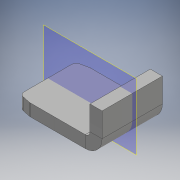
# Autodesk Inventor part: hage
Saved by Autodesk Inventor 2018 (Build 220112000, 112)
## iProperties
Created: 2019-09-30
Part Number: hage
Material: Steel
Document SubType Name: Sheet Metal
Designer: gust3763
Density: 7.85 g/cm^3
Sheet Metal Rule: Default_mm
Appearance: Light Gray
Mass: 86.5098 g
Surface Area: 39.7038 cm^2
Volume: 11.0204 cm^3
Author: gust3763
Autodesk Inventor part; units mm, degrees
ref_plane "YZ Plane" through (0, 0, 0) normal (1, 0, 0) x (0, 1, 0)
ref_plane "XZ Plane" through (0, 0, 0) normal (0, 1, 0) x (-1, 0, 0)
ref_plane "XY Plane" through (0, 0, 0) normal (0, 0, 1) x (1, 0, 0)
sketch "Sketch1" plane through (0, 0, 0) normal (0, 0, 1) x (1, 0, 0)
  line L0 (4.3681, -1.3047) -> (34.1579, -1.3047)
  line L1 (34.1579, -1.3047) -> (34.1579, 23.6953)
  line L2 (34.1579, 23.6953) -> (4.3681, 23.6953)
  line L3 (-0.8421, 21.0129) -> (-0.8421, 1.3776)
  line L4 (3.9523, 23.6516) -> (0.7421, 22.9692)
  line L5 (3.9523, -1.261) -> (0.7421, -0.5787)
  line L6 (4.1579, 23.6953) -> (4.1579, -1.3047) construction
  arc A0 (0.7421, 22.9692) -> (-0.8421, 21.0129) centre (1.1579, 21.0129) ccw
  arc A1 (-0.8421, 1.3776) -> (0.7421, -0.5787) centre (1.1579, 1.3776) ccw
  arc A2 (4.3681, 23.6953) -> (3.9523, 23.6516) centre (4.3681, 21.6953) ccw
  arc A3 (3.9523, -1.261) -> (4.3681, -1.3047) centre (4.3681, 0.6953) ccw
  point P0 (0, 0)
  point P1 (-0.8421, 22.6325)
  point P2 (-0.8421, -0.242)
  dimension "d3" = 12
  dimension "d4" = 25
  dimension "d5" = 12
  dimension "d7" = 35
  dimension "d8" = 5
  dimension "d20" = 2
  measures "d3" angle of L0 L5
  measures "d4" distance between parallel lines of L0 L2
  measures "d5" angle of L4 L2
  measures "d7" distance between parallel lines of L1 L3
  measures "d8" distance between parallel lines of L3 L6
  measures "d20" radius of A0
extrude "Plate1" add sketch "Sketch1" along normal blind 5
sketch "Sketch2" plane through (29.1579, 23.6953, 0) normal (1, 0, 0) x (0, 1, 0)
  line L0 (-25, 0) -> (0, 0)
  line L1 (0, 0) -> (0, 17)
  line L2 (0, 17) -> (-25, 17)
  line L3 (-25, 17) -> (-25, 0)
  constraints: 6 end point, 1 horizontal, 1 perpendicular, 1 vertical
edge flange "Flange1" height 12 angle 90 thickness 5 bend radius 2 thickness toward (1, 0, 0) relief straight relief width 5 relief depth 2.5 edges at (34.1579, 11.1953, 5) wall of the first edge with corners at (29.1579, -1.3047, 0) (29.1579, 23.6953, 0) (29.1579, 23.6953, 17) (29.1579, -1.3047, 17)
bend "Bend1"
corner "Corner1"
ref_plane "midtplan" through (4.3681, 11.1953, 5) normal (0, 1, 0) x (1, 0, 0)
equation "\"d3\" = d5"
equation "\"d9\" = Thickness"
equation "\"d10\" = BendReliefWidth"
equation "\"d11\" = BendReliefDepth"
equation "\"d12\" = MinimumRemnant"
equation "\"d13\" = TransitionRadius"
equation "\"d16\" = BendRadius"
equation "\"d17\" = CornerReliefSize"
equation "\"d18\" = GapSize"
equation "\"d19\" = JacobiRadiusSize"
equation "\"BendReliefWidth\" = Thickness"
equation "\"BendReliefDepth\" = 0.5 * Thickness"
equation "\"TransitionRadius\" = BendRadius"
equation "\"JacobiRadiusSize\" = BendRadius"
equation "\"GapSize\" = Thickness"
equation "\"Thickness\" = 5"
equation "\"MinimumRemnant\" = 10"
equation "\"BendRadius\" = 2"
equation "\"CornerReliefSize\" = 20"
body "Solid1"
